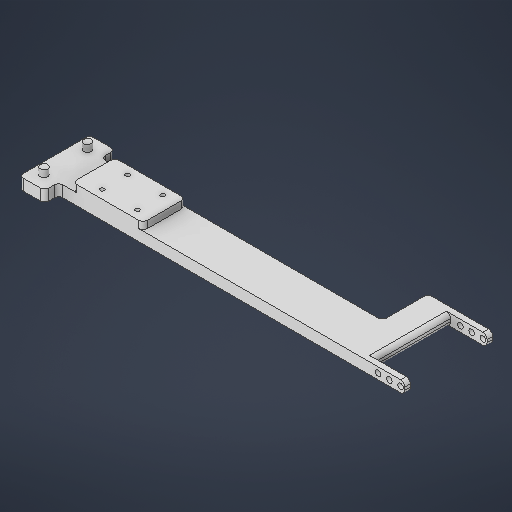
# Autodesk Inventor part: Arm
Saved by Autodesk Inventor 2026.1 (Build 301233020, 233B)
## iProperties
Created: 2025-10-26
Part Number: Arm
Material: Generic
Document SubType Name: Modeling
Designer: Garfieldcmix
Density: 1 g/cm^3
Appearance: Default
Author: Garfieldcmix
Autodesk Inventor part; units mm, degrees
ref_plane "YZ Plane" through (0, 0, 0) normal (1, 0, 0) x (0, 1, 0)
ref_plane "XZ Plane" through (0, 0, 0) normal (0, 1, 0) x (-1, 0, 0)
ref_plane "XY Plane" through (0, 0, 0) normal (0, 0, 1) x (1, 0, 0)
sketch "Sketch1" plane through (0, 0, 0) normal (0, 1, 0) x (-1, 0, 0)
  line L0 (8, 25) -> (8, -25)
  line L1 (8, -25) -> (-10, -25)
  line L2 (-10, -25) -> (-10, -15)
  line L3 (-10, -15) -> (-230, -15)
  line L4 (-230, -15) -> (-230, 15)
  line L5 (-230, 15) -> (-10, 15)
  line L6 (-10, 15) -> (-10, 25)
  line L7 (-10, 25) -> (8, 25)
  line L8 (55.6, 0) -> (-277.6, 0) construction
  point P0 (0, 0)
  dimension "d0" = 50
  dimension "d2" = 8
  dimension "d3" = 10
  dimension "d4" = 30
  dimension "d5" = 220
  constraints: 16 end point, 4 symmetric about line, 3 perpendicular, 1 vertical
  measures "d0" distance of L0.start L0.end
  measures "d2" horizontal distance of point (0, 0) L0.end
  measures "d3" horizontal distance of L1.end point (0, 0)
  measures "d4" distance of L3.end L4.end
  measures "d5" distance of L2.end L3.end
extrude "Extrusion1" add sketch "Sketch1" along normal blind 8
sketch "Sketch2" plane through (0, 8, 0) normal (0, 1, 0) x (1, 0, 0)
  circle A0 centre (0, -15.5) radius 2.75
  circle A1 centre (0, 15.5) radius 2.75
  line L0 (0, 35) -> (0, -35) construction
  line L1 (-55.6, 0) -> (277.6, 0) construction
  point P0 (0, 0)
  dimension "d8" = 5.5
  dimension "d9" = 31
  constraints: 2 centre point, 2 point on line, 1 equal radius, 1 symmetric about line
  measures "d8" diameter of A0
  measures "d9" distance of A1.centre A0.centre
extrude "Extrusion2" add sketch "Sketch2" along normal blind 4.9
sketch "Sketch3" plane through (0, 8, 0) normal (0, 1, 0) x (1, 0, 0)
  line L0 (230, 15) -> (10, 15) construction
  line L1 (10, -15) -> (230, -15) construction
  line L2 (20, 15) -> (70, 15)
  line L3 (70, 15) -> (70, -15)
  line L4 (70, -15) -> (20, -15)
  line L5 (20, -15) -> (20, 15)
  point P0 (0, 0)
  dimension "d12" = 10
  dimension "d13" = 50
  constraints: 8 end point, 2 parallel, 2 point on line, 1 horizontal, 1 perpendicular
  measures "d12" distance from line of L5 L0.end
  measures "d13" distance of L2.end L2.start
extrude "Extrusion3" add sketch "Sketch3" along normal blind 5.1
sketch "Sketch4" plane through (0, 13.1, 0) normal (0, 1, 0) x (1, 0, 0)
  circle A0 centre (35, 9) radius 1.475
  circle A1 centre (60, 9) radius 1.475
  circle A2 centre (35, -9) radius 1.475
  circle A3 centre (60, -9) radius 1.475
  line L0 (-55.6, 0) -> (277.6, 0) construction
  line L1 (35, 9) -> (35, -9) construction
  line L2 (60, 9) -> (60, -9) construction
  line L3 (20, 15) -> (20, -15) construction
  point P0 (0, 0)
  dimension "d16" = 2.95
  dimension "d17" = 18
  dimension "d18" = 25
  dimension "d19" = 15
  constraints: 4 centre point, 4 end point, 3 equal radius, 2 symmetric about line, 2 vertical, 1 parallel
  measures "d16" diameter of A0
  measures "d17" distance of L1.start L1.end
  measures "d18" distance of L2.start L1.start
  measures "d19" distance from line of L3 L1.start
extrude "Extrusion4" cut sketch "Sketch4" against normal up to surface (13.1 mm away)
sketch "Sketch7" plane through (230, 0, -15) normal (0, 0, -1) x (-1, 0, 0)
  line L0 (0, 0) -> (0, 8) projected
  line L1 (0, 8) -> (160, 8) projected
  line L2 (0, 0) -> (220, 0) projected
  line L3 (20, 0) -> (20, 8)
  point P0 (230, 0)
  dimension "d37" = 20
  constraints: 2 end point, 2 point on line, 1 perpendicular
  measures "d37" distance between parallel lines of L0 L3
extrude "Extrusion7" add sketch "Sketch7" along normal blind 32.5
sketch "Sketch8" plane through (230, 0, 15) normal (1, 0, 0) x (0, 0, -1)
  line L0 (0, 0) -> (0, 8) projected
  line L1 (62.5, 8) -> (62.5, 0) projected
  line L2 (0, 0) -> (62.5, 0) projected
  line L3 (0, 8) -> (62.5, 8) projected
  line L4 (4, 8) -> (4, 0)
  line L5 (58.5, 8) -> (58.5, 0)
  point P0 (15, 0)
  dimension "d40" = 4
  dimension "d41" = 4
  constraints: 4 end point, 4 point on line, 2 perpendicular
  measures "d40" distance between parallel lines of L0 L4
  measures "d41" distance between parallel lines of L1 L5
extrude "Extrusion8" add sketch "Sketch8" along normal blind 26 contours L0 L3 L4 L2 | L5 L3 L1 L2
sketch "Sketch9" plane through (10, 0, 15) normal (0, 0, 1) x (1, 0, 0)
  line L0 (246, 8) -> (246, 0) construction
  line L1 (246, 4) -> (227, 4) construction
  circle A0 centre (227, 4) radius 2
  circle A1 centre (235, 4) radius 2
  circle A2 centre (243, 4) radius 2
  point P0 (-10, 0)
  dimension "d44" = 4
  dimension "d45" = 8
  dimension "d46" = 8
  dimension "d47" = 3
  constraints: 3 centre point, 2 end point, 2 equal radius, 2 point on line, 1 coincident, 1 horizontal, 1 midpoint
  measures "d44" diameter of A0
  measures "d45" distance of A1.centre L1.end
  measures "d46" distance of A2.centre A1.centre
  measures "d47" distance from line of L0 A2.centre
extrude "Extrusion9" cut sketch "Sketch9" against normal up to surface (62.5 mm away)
fillet "Fillet4" radius 3 2 edges at (210, 4, -15) (210, 4, -47.5)
fillet "Fillet5" radius 3 6 edges at (230, 0, -16.25) (230, 8, -16.25) (256, 0, 13) (256, 8, 13) (256, 0, -45.5) (256, 8, -45.5)
fillet "Fillet2" radius 3 4 edges at (20, 10.55, 15) (20, 10.55, -15) (70, 10.55, 15) (70, 10.55, -15)
fillet "Fillet3" radius 3 6 edges at (10, 4, 15) (10, 4, 25) (-8, 4, 25) (-8, 4, -25) (10, 4, -25) (10, 4, -15)
body "Solid1"
